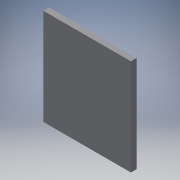
# Autodesk Inventor part: Ramp
Saved by Autodesk Inventor 2018 (Build 220112000, 112)
## iProperties
Created: 2018-01-12
Part Number: Ramp
Material: Generic
Document SubType Name: Modeling
Designer: Apple
Density: 1 g/cm^3
Appearance: Default
Author: Apple
Autodesk Inventor part; units mm, degrees
ref_plane "YZ Plane" through (0, 0, 0) normal (1, 0, 0) x (0, 1, 0)
ref_plane "XZ Plane" through (0, 0, 0) normal (0, 1, 0) x (-1, 0, 0)
ref_plane "XY Plane" through (0, 0, 0) normal (0, 0, 1) x (1, 0, 0)
sketch "Sketch1" plane through (0, 0, 0) normal (0, 0, 1) x (1, 0, 0)
  line L0 (-684.3164, 752.8778) -> (684.3164, 752.8778)
  line L1 (684.3164, 752.8778) -> (684.3164, -752.8778)
  line L2 (684.3164, -752.8778) -> (-684.3164, -752.8778)
  line L3 (-684.3164, -752.8778) -> (-684.3164, 752.8778)
  line L4 (-684.3164, 752.8778) -> (684.3164, -752.8778) construction
  line L5 (684.3164, 752.8778) -> (-684.3164, -752.8778) construction
  point P0 (0, 0)
  constraints: 12 end point, 2 midpoint, 2 parallel, 1 horizontal, 1 perpendicular
extrude "Extrusion1" add sketch "Sketch1" along normal blind 88.9
body "Solid1"
